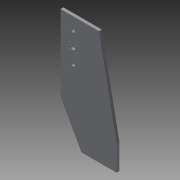
# Autodesk Inventor part: CNC-Y-axis- side plates with stepper
Saved by Autodesk Inventor 2015 (Build 190159000, 159)
## iProperties
Created: 2015-03-24
Part Number: CNC-Y-axis- side plates with stepper
Material: Generic
Document SubType Name: Modeling
Designer: Bangladesh
Density: 1 g/cm^3
Appearance: Default
Author: Bangladesh
Autodesk Inventor part; units mm, degrees
ref_plane "YZ Plane" through (0, 0, 0) normal (1, 0, 0) x (0, 1, 0)
ref_plane "XZ Plane" through (0, 0, 0) normal (0, 1, 0) x (-1, 0, 0)
ref_plane "XY Plane" through (0, 0, 0) normal (0, 0, 1) x (1, 0, 0)
sketch "Sketch1" plane through (0, 0, 0) normal (0, 0, 1) x (1, 0, 0)
  line L0 (-127.68, 259.036) -> (-127.68, -85.275)
  line L1 (-127.68, 259.036) -> (47.477, 259.036)
  line L2 (127.68, -259.036) -> (-32.32, -259.036)
  line L3 (-32.32, -259.036) -> (-127.68, -85.275)
  line L4 (127.68, -259.036) -> (127.68, -145.836)
  line L5 (127.68, -145.836) -> (47.477, 259.036)
  point P0 (0, 0)
  dimension "d6" = 344.311
  dimension "d7" = 175.157
  dimension "d9" = 160
  dimension "d10" = 113.2
  constraints: 12 end point, 1 horizontal
  measures "d6" distance of L0.start L0.end
  measures "d7" distance of L0.start L1.end
  measures "d9" distance of L2.start L2.end
  measures "d10" distance of L2.start L4.end
extrude "Extrusion1" add sketch "Sketch1" along normal mid plane 13
sketch "Sketch2" plane through (0, 0, 6.5) normal (0, 0, 1) x (1, 0, 0)
  circle A0 centre (-71.723, 203.108) radius 9
  circle A1 centre (-71.723, 69.504) radius 9
  circle A2 centre (-71.723, 136.306) radius 11
  line L0 (-87.483, 152.066) -> (-55.963, 152.066)
  line L1 (-55.963, 152.066) -> (-55.963, 120.546)
  line L2 (-55.963, 120.546) -> (-87.483, 120.546)
  line L3 (-87.483, 120.546) -> (-87.483, 152.066)
  line L4 (-87.483, 152.066) -> (-55.963, 120.546) construction
  line L5 (-55.963, 152.066) -> (-87.483, 120.546) construction
  circle A3 centre (-87.483, 152.066) radius 2.95
  circle A4 centre (-55.963, 152.066) radius 2.95
  circle A5 centre (-55.963, 120.546) radius 2.95
  circle A6 centre (-87.483, 120.546) radius 2.95
  line L6 (47.477, 259.036) -> (-127.68, 259.036) projected
  line L7 (-127.68, 259.036) -> (-127.68, -85.275) projected
  point P0 (0, 0)
  point P1 (-71.723, 136.306)
  dimension "d25" = 22
  dimension "d26" = 66.802
  dimension "d31" = 31.52
  dimension "d32" = 31.52
  dimension "d35" = 5.9
  dimension "d39" = 66.802
  dimension "d40" = 55.928
  dimension "d41" = 55.957
  dimension "d42" = 5.9
  constraints: 12 end point, 7 centre point, 4 coincident, 3 midpoint, 2 parallel, 2 vertical alignment, 1 horizontal, 1 perpendicular
  measures "d25" diameter of A2
  measures "d26" distance of A1.centre A2.centre
  measures "d31" distance of L1.end L2.end
  measures "d32" distance of L0.end L1.end
  measures "d35" diameter of A5
  measures "d39" distance of A0.centre A2.centre
  measures "d40" distance from line of L6 A0.centre
  measures "d41" distance from line of L7 A0.centre
  measures "d42" diameter of A6
extrude "Extrusion3" cut sketch "Sketch2" against normal blind 25.4 contours A0 | A1 | A2 | L3 A3 L0 | L0 A3 L3 | A4 L1 L0 | L0 L1 A4 | A6 L2 L3 | L3 L2 A6 | A5 L2 L1 | L1 L2 A5
equation "\"d32\" = d31"
body "Solid1"
